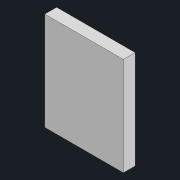
# Autodesk Inventor part: finger_1
Saved by Autodesk Inventor 2021 (Build 250183000, 183)
## iProperties
Created: 2021-07-10
Part Number: finger_1
Material: 一般
Document SubType Name: Modeling
Designer: yuta0
Density: 1 g/cm^3
Appearance: 既定
Author: yuta0
Autodesk Inventor part; units mm, degrees
ref_plane "YZ Plane" through (0, 0, 0) normal (1, 0, 0) x (0, 1, 0)
ref_plane "XZ Plane" through (0, 0, 0) normal (0, 1, 0) x (-1, 0, 0)
ref_plane "XY Plane" through (0, 0, 0) normal (0, 0, 1) x (1, 0, 0)
sketch "スケッチ1" plane through (0, 0, 0) normal (0, 1, 0) x (-1, 0, 0)
  line L0 (-20, 0) -> (20, 0)
  line L1 (20, 0) -> (20, -6)
  line L2 (20, -6) -> (-20, -6)
  line L3 (-20, -6) -> (-20, 0)
  line L4 (-20, 0) -> (20, -6) construction
  line L5 (20, 0) -> (-20, -6) construction
  point P0 (0, -3)
  point P1 (0, 0)
  dimension "d0" = 40
  dimension "d1" = 6
  dimension "d6" = 0
  dimension "d7" = 0
  constraints: 12 end point, 2 midpoint, 2 parallel, 1 horizontal, 1 perpendicular
  measures "d0" distance of L0.start L0.end
  measures "d1" distance of L0.end L1.end
  measures "d6" distance from line of point (0, 0) L0
  measures "d7" horizontal distance of point (0, 0) point (0, -3)
extrude "押し出し1" add sketch "スケッチ1" along normal blind 50
